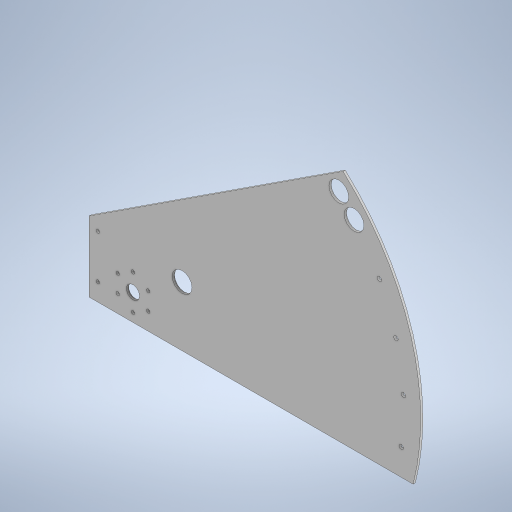
# Autodesk Inventor part: Shooter Side
Saved by Autodesk Inventor 2023.3 (Build 273359000, 359)
## iProperties
Created: 2023-10-19
Part Number: Shooter Side
Material: Generic
Document SubType Name: Modeling
Designer: jackc
Density: 1 g/cm^3
Appearance: Default
Author: jackc
Autodesk Inventor part; units mm, degrees
ref_plane "YZ Plane" through (0, 0, 0) normal (1, 0, 0) x (0, 1, 0)
ref_plane "XZ Plane" through (0, 0, 0) normal (0, 1, 0) x (-1, 0, 0)
ref_plane "XY Plane" through (0, 0, 0) normal (0, 0, 1) x (1, 0, 0)
sketch "Sketch1" plane through (0, 0, 0) normal (0, 0, 1) x (1, 0, 0)
  line L0 (0, 0) -> (468.8863, 0)
  line L1 (0, 0) -> (0, 101.6)
  line L2 (0, 101.6) -> (367.4132, 341.2775)
  arc A0 (468.8863, 0) -> (367.4132, 341.2775) centre (134.655, 86.3463) ccw
  circle A1 centre (134.655, 86.3463) radius 14.2875
  circle A2 centre (361.4065, 313.0978) radius 20.6375 construction
  circle A3 centre (134.655, 86.3463) radius 50.8 construction
  circle A4 centre (63.5, 37.85) radius 9.525
  circle A5 centre (361.4065, 313.0978) radius 14.2875
  arc A6 (443.4863, 0) -> (346.1395, 327.3998) centre (134.655, 86.3463) ccw construction
  line L3 (134.655, 86.3463) -> (361.4065, 313.0978) construction
  circle A7 centre (63.5, 37.85) radius 31.5 construction
  circle A8 centre (383.5221, 288.578) radius 14.2875
  circle A9 centre (12.7, 88.9) radius 2.4892
  circle A10 centre (12.7, 25.4) radius 2.4892
  circle A11 centre (419.9711, 232.7267) radius 3.175
  circle A12 centre (444.079, 170.544) radius 3.175
  circle A13 centre (451.6799, 38.1) radius 3.175
  circle A14 centre (454.8033, 104.7193) radius 3.175
  line L4 (383.5221, 288.578) -> (419.9711, 232.7267) construction
  line L5 (419.9711, 232.7267) -> (444.079, 170.544) construction
  line L6 (454.8033, 104.7193) -> (444.079, 170.544) construction
  line L7 (451.6799, 38.1) -> (454.8033, 104.7193) construction
  circle A15 centre (63.5, 63.25) radius 2.4892
  circle A16 centre (41.503, 50.55) radius 2.4892
  circle A17 centre (41.503, 25.15) radius 2.4892
  circle A18 centre (63.5, 12.45) radius 2.4892
  circle A19 centre (85.497, 25.15) radius 2.4892
  circle A20 centre (85.497, 50.55) radius 2.4892
  point P0 (0, 50.8)
  dimension "d0" = 28.575
  dimension "d1" = 41.275
  dimension "d2" = 101.6
  dimension "d3" = 19.05
  dimension "d5" = 28.575
  dimension "d6" = 320.675
  dimension "d7" = 25.4
  dimension "d8" = 25.4
  dimension "d9" = 45
  dimension "d10" = 63
  dimension "d11" = 33.02
  dimension "d12" = 20.32
  dimension "d13" = 4.9784
  dimension "d14" = 12.7
  dimension "d15" = 63.5
  dimension "d16" = 25.4
  dimension "d17" = 86.11
  dimension "d18" = 37.85
  dimension "d19" = 12.7
  dimension "d20" = 6.35
  dimension "d21" = 38.1
  dimension "d22" = 63.5
  dimension "d23" = 25.4
  dimension "d26" = 360
  constraints: 21 centre point, 16 end point, 10 point on circle, 6 equal radius, 4 coincident, 3 equal length, 2 point on line, 2 vertical alignment, 1 concentric, 1 horizontal, 1 midpoint, 1 vertical, 13 other
  measures "d0" diameter of A1
  measures "d1" diameter of A2
  measures "d2" diameter of A3
  measures "d3" diameter of A4
  measures "d5" diameter of A5
  measures "d6" distance of A0.centre A2.centre
  measures "d7" distance of L2.end A6.end
  measures "d8" distance of L0.end A6.start
  measures "d9" angle of L0 L3
  measures "d10" diameter of A7
  measures "d11" distance of A2.centre L4.start
  measures "d12" distance from line of L2 L3.end
  measures "d13" diameter of A9
  measures "d14" distance from line of A9.centre L1
  measures "d15" distance of A9.centre A10.centre
  measures "d16" distance from line of A10.centre L0
  measures "d17" distance of A3.centre A7.centre
  measures "d18" distance from line of A4.centre L0
  measures "d19" horizontal distance of L1.end A9.centre
  measures "d20" diameter of A11
  measures "d21" distance from line of L0 L7.start
  measures "d22" horizontal distance of A4.centre point (0, 50.8)
  measures "d23" distance of A15.centre A7.centre
extrude "Extrusion1" add sketch "Sketch1" along normal blind 3.175
equation "\"d2\" = WheelSize"
equation "\"d5\" = d0"
equation "\"d6\" = d1 + BallSize + 0.5 * WheelSize - Compression"
equation "\"d8\" = d7"
equation "\"WheelSize\" = 101.6"
equation "\"BallSize\" = 241.3"
equation "\"Compression\" = 12.7"
body "Solid1"
